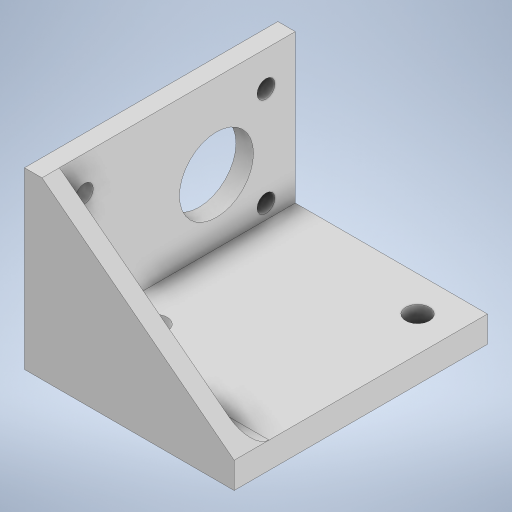
# Autodesk Inventor part: Motor Mount V1
Saved by Autodesk Inventor 2024.2 (Build 282272000, 272)
## iProperties
Created: 2024-07-25
Part Number: Motor Mount V1
Material: Generic
Document SubType Name: Modeling
Designer: balmo
Density: 1 g/cm^3
Appearance: Default
Author: balmo
## iProperties of the stored document Motor Mount V1_3DPrint.ipt
Created: 2024-07-25
Part Number: Motor Mount V1_3DPrint
Material: Generic
Document SubType Name: Modeling
Designer: balmo
Density: 1 g/cm^3
Appearance: Default
Author: balmo
Autodesk Inventor part; units mm, degrees
ref_plane "YZ Plane" through (0, 0, 0) normal (1, 0, 0) x (0, 1, 0)
ref_plane "XZ Plane" through (0, 0, 0) normal (0, 1, 0) x (-1, 0, 0)
ref_plane "XY Plane" through (0, 0, 0) normal (0, 0, 1) x (1, 0, 0)
sketch "Sketch1" plane through (0, 0, 0) normal (0, 1, 0) x (-1, 0, 0)
  line L0 (0, 0) -> (31.75, 0)
  line L1 (31.75, 0) -> (31.75, -3.175)
  line L2 (31.75, -3.175) -> (4.7625, -3.175)
  line L3 (4.7625, -3.175) -> (4.7625, -38.1)
  line L4 (4.7625, -38.1) -> (0, -38.1)
  line L5 (0, 0) -> (0, -38.1)
  point P0 (31.75, -1.5875)
  dimension "d1" = 3.175
  dimension "d2" = 31.75
  dimension "d3" = 38.1
  dimension "d4" = 4.7625
  constraints: 12 end point, 1 horizontal, 1 midpoint, 1 parallel, 1 perpendicular, 1 vertical
  measures "d1" distance between parallel lines of L0 L2
  measures "d2" distance from line of L5 point (31.75, -1.587)
  measures "d3" distance between parallel lines of L4 L0
  measures "d4" distance between parallel lines of L5 L3
extrude "Extrusion1" add sketch "Sketch1" along normal blind 46.0375
sketch "Sketch2" plane through (-31.75, 0, 0) normal (0, 0, 1) x (1, 0, 0)
  line L0 (0, 0) -> (0, 46.0375) projected
  line L1 (31.75, 0) -> (31.75, 46.0375) projected
  line L2 (6.35, 5.334) -> (24.35, 5.334) construction
  line L3 (24.35, 5.334) -> (24.35, 38.334) construction
  line L4 (24.35, 38.334) -> (6.35, 38.334) construction
  line L5 (6.35, 38.334) -> (6.35, 5.334) construction
  circle A0 centre (6.35, 5.334) radius 1.625
  circle A1 centre (24.35, 5.334) radius 1.625
  circle A2 centre (6.35, 38.334) radius 1.625
  circle A3 centre (24.35, 38.334) radius 1.625
  line L6 (0, 0) -> (31.75, 0) projected
  circle A4 centre (15.35, 14.334) radius 6.731
  circle A5 centre (24.35, 5.334) radius 2.25
  dimension "d23" = 3.25
  dimension "d24" = 3.25
  dimension "d25" = 3.25
  dimension "d26" = 3.25
  dimension "d27" = 33
  dimension "d28" = 18
  dimension "d33" = 6.35
  dimension "d34" = 5.334
  dimension "d37" = 9
  dimension "d38" = 13.462
  dimension "d52" = 4.5
  constraints: 8 end point, 6 centre point, 5 coincident, 2 parallel, 1 horizontal, 1 perpendicular
  measures "d23" diameter of A0
  measures "d24" diameter of A1
  measures "d25" diameter of A2
  measures "d26" diameter of A3
  measures "d27" distance between parallel lines of L4 L2
  measures "d28" distance between parallel lines of L5 L3
  measures "d33" distance from line of L0 A0.centre
  measures "d34" distance between parallel lines of L6 L2
  measures "d37" horizontal distance of A4.centre A0.centre
  measures "d38" diameter of A4
  measures "d52" diameter of A5
extrude "Extrusion2" cut sketch "Sketch2" against normal blind 46.0375 contours A0 | A1 | A2 | A3 | A4
sketch "Sketch3" plane through (0, 46.0375, 0) normal (0, 1, 0) x (1, 0, 0)
  line L0 (0, 38.1) -> (-4.7625, 38.1) projected
  line L1 (-4.7625, 38.1) -> (-4.7625, 3.175) projected
  line L2 (-4.7625, 3.175) -> (-31.75, 3.175) projected
  line L3 (-31.75, 3.175) -> (-31.75, 0) projected
  line L4 (-31.75, 0) -> (0, 0) projected
  line L5 (0, 0) -> (0, 38.1) projected
  line L6 (-31.75, 3.175) -> (-4.7625, 38.1)
  constraints: 2 end point
extrude "Extrusion3" add sketch "Sketch3" against normal blind 3.175 contours L1 L2 L6
sketch "Sketch4" plane through (-4.7625, 0, -38.1) normal (-1, 0, 0) x (0, 0, 1)
  circle A0 centre (28.575, 31.75) radius 2.159
  circle A1 centre (6.35, 6.35) radius 2.159
  line L0 (0, 0) -> (0, 42.8625) projected
  line L1 (0, 0) -> (34.925, 0) projected
  line L2 (34.925, 42.8625) -> (0, 42.8625) projected
  line L3 (34.925, 0) -> (34.925, 42.8625) projected
  circle A2 centre (28.575, 31.75) radius 4.3656
  point P0 (38.1, 0)
  dimension "d41" = 4.318
  dimension "d42" = 4.318
  dimension "d43" = 6.35
  dimension "d44" = 6.35
  dimension "d45" = 11.1125
  dimension "d47" = 6.35
  dimension "d50" = 8.7312
  constraints: 3 centre point, 1 coincident
  measures "d41" diameter of A0
  measures "d42" diameter of A1
  measures "d43" distance from line of A1.centre L0
  measures "d44" distance from line of A1.centre L1
  measures "d45" distance from line of L2 A0.centre
  measures "d47" distance from line of L3 A0.centre
  measures "d50" diameter of A2
extrude "Extrusion4" cut sketch "Sketch4" against normal through all contours A0 | A1
fillet "Fillet1" radius 3.175 1 edges at (-4.7625, 42.8625, -20.6375)
body "Solid1"
